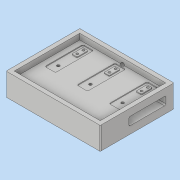
# Autodesk Inventor part: Hauptplatte
Saved by Autodesk Inventor 2018 (Build 220112000, 112)
## iProperties
Created: 2020-10-04
Part Number: Hauptplatte
Material: Generisch
Document SubType Name: Modeling
Designer: marce
Density: 1 g/cm^3
Appearance: Vorgabe
Author: marce
Autodesk Inventor part; units mm, degrees
ref_plane "YZ Plane" through (0, 0, 0) normal (1, 0, 0) x (0, 1, 0)
ref_plane "XZ Plane" through (0, 0, 0) normal (0, 1, 0) x (-1, 0, 0)
ref_plane "XY Plane" through (0, 0, 0) normal (0, 0, 1) x (1, 0, 0)
sketch "Skizze1" plane through (0, 0, 0) normal (0, 0, 1) x (1, 0, 0)
  line L0 (0, 0) -> (230, 0)
  line L1 (230, 0) -> (230, 180)
  line L2 (230, 180) -> (0, 180)
  line L3 (0, 180) -> (0, 0)
  dimension "d0" = 230
  dimension "d1" = 180
  constraints: 8 end point, 2 parallel, 1 horizontal, 1 perpendicular
  measures "d0" distance of L2.end L1.end
  measures "d1" distance of L1.end L0.end
extrude "Extrusion1" add sketch "Skizze1" along normal blind 39
sketch "Skizze2" plane through (0, 0, 39) normal (0, 0, 1) x (1, 0, 0)
  line L0 (0, 0) -> (230, 0) projected
  line L1 (230, 0) -> (230, 180) projected
  line L2 (230, 180) -> (0, 180) projected
  line L3 (0, 180) -> (0, 0) projected
  line L4 (10, 170) -> (220, 170)
  line L5 (220, 170) -> (220, 10)
  line L6 (220, 10) -> (10, 10)
  line L7 (10, 10) -> (10, 170)
  dimension "d4" = 10
  constraints: 8 end point, 3 other
  measures "d4" distance between parallel lines of L2 L4
extrude "Extrusion2" add sketch "Skizze2" along normal blind 16
sketch "Skizze3" plane through (0, 0, 39) normal (0, 0, 1) x (1, 0, 0)
  line L0 (108.5, 157.5) -> (121.5, 157.5)
  line L1 (121.5, 157.5) -> (121.5, 130.5)
  line L2 (121.5, 130.5) -> (108.5, 130.5)
  line L3 (108.5, 130.5) -> (108.5, 157.5)
  line L4 (30, 157.5) -> (43, 157.5)
  line L5 (43, 157.5) -> (43, 130.5)
  line L6 (43, 130.5) -> (30, 130.5)
  line L7 (30, 130.5) -> (30, 157.5)
  line L8 (187, 157.5) -> (200, 157.5)
  line L9 (200, 157.5) -> (200, 130.5)
  line L10 (200, 130.5) -> (187, 130.5)
  line L11 (187, 130.5) -> (187, 157.5)
  line L12 (10, 170) -> (10, 10) projected
  line L13 (220, 10) -> (220, 170) projected
  line L14 (220, 170) -> (10, 170) projected
  line L15 (23.5, 164) -> (49.5, 164)
  line L16 (49.5, 164) -> (49.5, 71)
  line L17 (49.5, 71) -> (23.5, 71)
  line L18 (23.5, 71) -> (23.5, 164)
  line L19 (102, 164) -> (128, 164)
  line L20 (128, 164) -> (128, 71)
  line L21 (128, 71) -> (102, 71)
  line L22 (102, 71) -> (102, 164)
  line L23 (180.5, 164) -> (206.5, 164)
  line L24 (206.5, 164) -> (206.5, 71)
  line L25 (206.5, 71) -> (180.5, 71)
  line L26 (180.5, 71) -> (180.5, 164)
  line L27 (220, 10) -> (220, 170) projected
  line L28 (220, 170) -> (10, 170) projected
  line L29 (10, 170) -> (10, 10) projected
  line L30 (10, 10) -> (220, 10) projected
  point P0 (0, 0)
  dimension "d7" = 27
  dimension "d8" = 13
  dimension "d9" = 27
  dimension "d10" = 13
  dimension "d11" = 27
  dimension "d12" = 13
  dimension "d13" = 20
  dimension "d14" = 20
  dimension "d15" = 65.5
  dimension "d16" = 65.5
  dimension "d17" = 12.5
  dimension "d34" = 6.5
  dimension "d35" = 6.5
  dimension "d36" = 6.5
  dimension "d37" = 6.5
  dimension "d38" = 6.5
  dimension "d39" = 6.5
  dimension "d40" = 6.5
  dimension "d42" = 93
  dimension "d43" = 93
  dimension "d44" = 93
  constraints: 48 end point, 12 parallel, 6 horizontal, 6 perpendicular, 3 collinear, 1 point on line
  measures "d7" distance of L0.end L1.end
  measures "d8" distance of L0.start L0.end
  measures "d9" distance of L4.end L5.end
  measures "d10" distance of L4.start L4.end
  measures "d11" distance of L8.end L9.end
  measures "d12" distance of L8.start L8.end
  measures "d13" distance between parallel lines of L7 L12
  measures "d14" distance between parallel lines of L13 L9
  measures "d15" distance between parallel lines of L11 L1
  measures "d16" distance between parallel lines of L5 L3
  measures "d17" distance between parallel lines of L14 L0
  measures "d34" distance between parallel lines of L18 L7
  measures "d35" distance between parallel lines of L16 L5
  measures "d36" distance between parallel lines of L3 L22
  measures "d37" distance between parallel lines of L20 L1
  measures "d38" distance between parallel lines of L26 L11
  measures "d39" distance between parallel lines of L24 L9
  measures "d40" distance between parallel lines of L23 L8
  measures "d42" distance of L21.end L19.start
  measures "d43" distance of L15.end L16.end
  measures "d44" distance of L25.end L23.start
extrude "Extrusion3" add sketch "Skizze3" along normal blind 2
sketch "Skizze4" plane through (0, 0, 41) normal (0, 0, 1) x (1, 0, 0)
  line L0 (43, 157.5) -> (30, 157.5) projected
  line L1 (30, 157.5) -> (30, 130.5) projected
  line L2 (30, 130.5) -> (43, 130.5) projected
  line L3 (43, 130.5) -> (43, 157.5) projected
  line L4 (121.5, 157.5) -> (108.5, 157.5) projected
  line L5 (108.5, 157.5) -> (108.5, 130.5) projected
  line L6 (108.5, 130.5) -> (121.5, 130.5) projected
  line L7 (121.5, 130.5) -> (121.5, 157.5) projected
  line L8 (200, 157.5) -> (187, 157.5) projected
  line L9 (187, 157.5) -> (187, 130.5) projected
  line L10 (187, 130.5) -> (200, 130.5) projected
  line L11 (200, 130.5) -> (200, 157.5) projected
  line L12 (30, 157.5) -> (36.5, 157.5)
  line L13 (36.5, 157.5) -> (36.5, 152.5)
  line L14 (36.5, 152.5) -> (30, 152.5)
  line L15 (30, 152.5) -> (30, 157.5)
  line L16 (36.5, 152.5) -> (50, 152.5)
  line L17 (50, 152.5) -> (50, 137.5)
  line L18 (50, 137.5) -> (36.5, 137.5)
  line L19 (36.5, 137.5) -> (36.5, 152.5)
  line L20 (115, 157.5) -> (120, 157.5)
  line L21 (120, 157.5) -> (120, 152.5)
  line L22 (120, 152.5) -> (115, 152.5)
  line L23 (115, 152.5) -> (115, 157.5)
  line L24 (115, 152.5) -> (121, 152.5)
  line L25 (121, 152.5) -> (121, 137.5)
  line L26 (121, 137.5) -> (115, 137.5)
  line L27 (115, 137.5) -> (115, 152.5)
  line L28 (200, 157.5) -> (187, 157.5) projected
  line L29 (193.5, 157.5) -> (198, 157.5)
  line L30 (198, 157.5) -> (198, 152.5)
  line L31 (198, 152.5) -> (193.5, 152.5)
  line L32 (193.5, 152.5) -> (193.5, 157.5)
  line L33 (193.5, 152.5) -> (200, 152.5)
  line L34 (200, 152.5) -> (200, 137.5)
  line L35 (200, 137.5) -> (193.5, 137.5)
  line L36 (193.5, 137.5) -> (193.5, 152.5)
  point P0 (0, 0)
  dimension "d20" = 15
  dimension "d21" = 5
  dimension "d29" = 5
  dimension "d30" = 15
  dimension "d31" = 5
  dimension "d32" = 15
  constraints: 48 end point, 12 parallel, 6 horizontal, 6 perpendicular, 3 midpoint, 1 point on line, 1 vertical alignment
  measures "d20" distance of L16.end L17.end
  measures "d21" distance of L12.end L13.end
  measures "d29" distance of L20.end L21.end
  measures "d30" distance of L24.end L25.end
  measures "d31" distance of L29.end L30.end
  measures "d32" distance of L33.end L34.end
hole "Bohrung1" at (36.5, 137.5, 41) at (36.5, 152.5, 41) at (115, 152.5, 41) at (115, 137.5, 41) at (193.5, 152.5, 41) at (193.5, 137.5, 41) direction (0, 0, -1) diameter 5.5 end through all
sketch "Skizze5" plane through (0, 0, 0) normal (0, 0, -1) x (-1, 0, 0)
  circle A0 centre (-193.5, 152.5) radius 2.75 projected
  circle A1 centre (-115, 152.5) radius 2.75 projected
  circle A2 centre (-36.5, 137.5) radius 2.75 projected
  circle A3 centre (-36.5, 152.5) radius 2.75 projected
  circle A4 centre (-115, 137.5) radius 2.75 projected
  circle A5 centre (-193.5, 137.5) radius 2.75 projected
  line L0 (0, 0) -> (-230, 0) projected
  line L1 (0, 180) -> (0, 0) projected
  line L2 (-230, 180) -> (0, 180) projected
  line L3 (-230, 0) -> (-230, 180) projected
  line L4 (-20, 160) -> (-20, 20)
  line L5 (-20, 20) -> (-210, 20)
  line L6 (-210, 20) -> (-210, 160)
  line L7 (-210, 160) -> (-20, 160)
  dimension "d46" = 20
  constraints: 8 end point, 3 other
  measures "d46" distance between parallel lines of L2 L7
extrude "Extrusion4" cut sketch "Skizze5" against normal blind 10 contours L4 L5 L6 L7
sketch "Skizze6" plane through (0, 0, 10) normal (0, 0, -1) x (-1, 0, 0)
  circle A0 centre (-193.5, 137.5) radius 2.75 projected
  circle A1 centre (-115, 137.5) radius 2.75 projected
  circle A2 centre (-36.5, 152.5) radius 2.75 projected
  circle A3 centre (-36.5, 137.5) radius 2.75 projected
  circle A4 centre (-115, 152.5) radius 2.75 projected
  circle A5 centre (-193.5, 152.5) radius 2.75 projected
  line L0 (-20, 160) -> (-20, 20) projected
  line L1 (-210, 160) -> (-20, 160) projected
  line L2 (-210, 20) -> (-210, 160) projected
  line L3 (-20, 20) -> (-210, 20) projected
  circle A6 centre (-193.5, 152.5) radius 2.75 projected
  circle A7 centre (-193.5, 152.5) radius 4.5
  circle A8 centre (-193.5, 137.5) radius 4.5
  circle A9 centre (-115, 152.5) radius 2.75 projected
  circle A10 centre (-115, 152.5) radius 4.5
  circle A11 centre (-115, 137.5) radius 4.5
  circle A12 centre (-36.5, 152.5) radius 2.75 projected
  circle A13 centre (-36.5, 152.5) radius 4.5
  circle A14 centre (-36.5, 137.5) radius 4.5
  point P0 (0, 0)
  dimension "d49" = 9
  dimension "d50" = 9
  dimension "d51" = 9
  dimension "d52" = 9
  dimension "d53" = 9
  dimension "d54" = 9
  constraints: 6 centre point, 6 coincident
  measures "d49" diameter of A7
  measures "d50" diameter of A8
  measures "d51" diameter of A10
  measures "d52" diameter of A11
  measures "d53" diameter of A13
  measures "d54" diameter of A14
extrude "Extrusion5" cut sketch "Skizze6" against normal blind 5.5 contours A7 | A8 | A10 | A11 | A13 | A14
sketch "Skizze7" plane through (0, 180, 0) normal (0, 1, 0) x (1, 0, 0)
  line L0 (230, 0) -> (0, 0) projected
  line L1 (0, 0) -> (0, -55) projected
  line L2 (230, -55) -> (0, -55) projected
  line L3 (230, 0) -> (230, -55) projected
  line L4 (230, -55) -> (0, -55)
  line L5 (0, -55) -> (0, -32)
  line L6 (0, -32) -> (230, -32)
  line L7 (230, -32) -> (230, -55)
  line L8 (115, -55) -> (101, -55)
  line L9 (101, -55) -> (101, -41)
  line L10 (101, -41) -> (115, -41)
  line L11 (115, -41) -> (115, -55)
  dimension "d59" = 14
  constraints: 16 end point, 4 parallel, 2 horizontal, 2 perpendicular, 1 midpoint, 1 point on line
  measures "d59" distance of L8.end L9.end
hole "Bohrung2" at (115, 180, 41) direction (0, -1, 0) diameter 10 depth 12 tip angle 118
sketch "Skizze8" plane through (0, 0, 0) normal (0, 0, -1) x (-1, 0, 0)
  line L0 (-210, 160) -> (-20, 160) projected
  line L1 (-20, 160) -> (-20, 20) projected
  line L2 (-20, 20) -> (-210, 20) projected
  line L3 (-210, 20) -> (-210, 160) projected
  line L4 (0, 0) -> (-230, 0) projected
  line L5 (0, 180) -> (0, 0) projected
  line L6 (-230, 180) -> (0, 180) projected
  line L7 (-230, 0) -> (-230, 180) projected
  line L8 (-10, 170) -> (-10, 10)
  line L9 (-10, 10) -> (-220, 10)
  line L10 (-220, 10) -> (-220, 170)
  line L11 (-220, 170) -> (-10, 170)
  dimension "d67" = 10
  dimension "d68" = 10
  constraints: 8 end point, 3 other
  measures "d67" distance between parallel lines of L6 L11
  measures "d68" distance between parallel lines of L0 L11
hole "Bohrung3" at (220, 170, 0) at (10, 170, 0) at (10, 10, 0) at (220, 10, 0) direction (0, 0, 1) diameter 6.647 depth 30 tip angle 118 thread size "M8x1.25" class "6H" standard "ISO Metric profile"
sketch "Skizze9" plane through (0, 0, 10) normal (0, 0, -1) x (-1, 0, 0)
  line L0 (-195, 121) -> (-35, 121)
  line L1 (-35, 121) -> (-35, 35)
  line L2 (-35, 35) -> (-195, 35)
  line L3 (-195, 35) -> (-195, 121)
  line L4 (-20, 160) -> (-20, 20) projected
  line L5 (-210, 20) -> (-210, 160) projected
  line L6 (-20, 20) -> (-210, 20) projected
  point P0 (0, 0)
  dimension "d76" = 15
  dimension "d77" = 15
  dimension "d78" = 15
  constraints: 8 end point, 2 parallel, 1 horizontal, 1 perpendicular
  measures "d76" distance between parallel lines of L4 L1
  measures "d77" distance between parallel lines of L5 L3
  measures "d78" distance between parallel lines of L6 L2
hole "Bohrung4" at (35, 121, 10) at (35, 35, 10) at (195, 35, 10) at (195, 121, 10) direction (0, 0, 1) diameter 6.647 depth 20 tip angle 118 thread size "M8x1.25" class "6H" standard "ISO Metric profile"
sketch "Skizze10" plane through (0, 0, 39) normal (0, 0, 1) x (1, 0, 0)
  line L0 (49.5, 71) -> (49.5, 164) projected
  line L1 (49.5, 164) -> (23.5, 164) projected
  line L2 (23.5, 164) -> (23.5, 71) projected
  line L3 (23.5, 71) -> (49.5, 71) projected
  line L4 (43, 157.5) -> (43, 130.5) projected
  line L5 (43, 130.5) -> (30, 130.5) projected
  line L6 (30, 130.5) -> (30, 157.5) projected
  line L7 (30, 157.5) -> (43, 157.5) projected
  line L8 (128, 71) -> (128, 164) projected
  line L9 (128, 164) -> (102, 164) projected
  line L10 (102, 164) -> (102, 71) projected
  line L11 (102, 71) -> (128, 71) projected
  line L12 (121.5, 157.5) -> (121.5, 130.5) projected
  line L13 (121.5, 130.5) -> (108.5, 130.5) projected
  line L14 (108.5, 130.5) -> (108.5, 157.5) projected
  line L15 (108.5, 157.5) -> (121.5, 157.5) projected
  line L16 (206.5, 71) -> (206.5, 164) projected
  line L17 (206.5, 164) -> (180.5, 164) projected
  line L18 (180.5, 164) -> (180.5, 71) projected
  line L19 (180.5, 71) -> (206.5, 71) projected
  line L20 (200, 157.5) -> (200, 130.5) projected
  line L21 (200, 130.5) -> (187, 130.5) projected
  line L22 (187, 130.5) -> (187, 157.5) projected
  line L23 (187, 157.5) -> (200, 157.5) projected
  line L24 (23.5, 71) -> (49.5, 71) projected
  line L25 (36.5, 71) -> (63, 71)
  line L26 (63, 71) -> (63, 91)
  line L27 (63, 91) -> (36.5, 91)
  line L28 (36.5, 91) -> (36.5, 71)
  line L29 (102, 71) -> (128, 71) projected
  line L30 (115, 71) -> (141, 71)
  line L31 (141, 71) -> (141, 91)
  line L32 (141, 91) -> (115, 91)
  line L33 (115, 91) -> (115, 71)
  line L34 (180.5, 71) -> (206.5, 71) projected
  line L35 (193.5, 71) -> (169, 71)
  line L36 (169, 71) -> (169, 91)
  line L37 (169, 91) -> (193.5, 91)
  line L38 (193.5, 91) -> (193.5, 71)
  point P0 (0, 0)
  dimension "d86" = 20
  constraints: 24 end point, 8 parallel, 3 horizontal, 3 midpoint, 3 perpendicular
  measures "d86" distance of L26.end L25.end
hole "Bohrung5" at (36.5, 91, 39) at (115, 91, 39) at (193.5, 91, 39) direction (0, 0, -1) diameter 6.647 end through all thread size "M8x1.25" class "6H" standard "ISO Metric profile"
sketch "Skizze11" plane through (0, 0, 10) normal (0, 0, -1) x (-1, 0, 0)
  circle A0 centre (-115, 91) radius 3.3235 projected
  circle A1 centre (-36.5, 91) radius 3.3235 projected
  circle A2 centre (-193.5, 91) radius 3.3235 projected
  circle A3 centre (-195, 35) radius 3.3235 projected
  circle A4 centre (-35, 121) radius 3.3235 projected
  circle A5 centre (-35, 35) radius 3.3235 projected
  circle A6 centre (-195, 121) radius 3.3235 projected
  circle A7 centre (-36.5, 152.5) radius 4.5 projected
  circle A8 centre (-115, 152.5) radius 4.5 projected
  circle A9 centre (-193.5, 152.5) radius 4.5 projected
  circle A10 centre (-193.5, 137.5) radius 4.5 projected
  circle A11 centre (-115, 137.5) radius 4.5 projected
  circle A12 centre (-36.5, 137.5) radius 4.5 projected
  line L0 (-20, 160) -> (-20, 20) projected
  line L1 (-210, 160) -> (-20, 160) projected
  line L2 (-210, 20) -> (-210, 160) projected
  line L3 (-20, 20) -> (-210, 20) projected
  circle A13 centre (-193.5, 91) radius 10
  circle A14 centre (-115, 91) radius 10
  circle A15 centre (-36.5, 91) radius 10
  point P0 (0, 0)
  dimension "d94" = 20
  constraints: 3 centre point, 3 coincident, 2 equal radius
  measures "d94" diameter of A13
extrude "Extrusion6" cut sketch "Skizze11" against normal blind 10 contours A13 | A14 | A15
sketch "Skizze12" plane through (230, 0, 0) normal (1, 0, 0) x (0, 0, -1)
  line L0 (-38, 70) -> (-18, 70)
  line L1 (-18, 70) -> (-18, 160)
  line L2 (-18, 160) -> (-38, 160)
  line L3 (-38, 160) -> (-38, 70)
  line L4 (0, 180) -> (-55, 180) projected
  line L5 (0, 0) -> (-55, 0) projected
  line L6 (0, 0) -> (0, 180) projected
  line L7 (-55, 0) -> (-55, 180) projected
  dimension "d99" = 90
  dimension "d100" = 20
  dimension "d101" = 20
  dimension "d102" = 70
  dimension "d103" = 18
  dimension "d104" = 17
  constraints: 8 end point, 2 parallel, 1 horizontal, 1 perpendicular
  measures "d99" distance of L2.end L0.start
  measures "d100" distance of L1.end L2.end
  measures "d101" distance between parallel lines of L4 L2
  measures "d102" distance between parallel lines of L5 L0
  measures "d103" distance between parallel lines of L6 L1
  measures "d104" distance between parallel lines of L3 L7
extrude "Extrusion7" cut sketch "Skizze12" against normal blind 25 contours L3 L2 L1 L0
fillet "Rundung3" radius 3.1 4 edges at (217.5, 70, 38) (217.5, 70, 18) (217.5, 160, 18) (217.5, 160, 38)
ref_plane "Arbeitsebene1" through (115, 0, 0) normal (1, 0, 0) x (0, 0, -1)
mirror "Spiegeln1" about plane through (115, 0, 0) normal (1, 0, 0) of "Rundung3", "Extrusion7"
fillet "Rundung2" radius 6.5 4 edges at (20, 160, 5) (210, 160, 5) (210, 20, 5) (20, 20, 5)
fillet "Rundung2" radius 2 4 edges at (230, 0, 27.5) (0, 0, 27.5) (0, 180, 27.5) (230, 180, 27.5)
fillet "Rundung1" radius 2 12 edges at (187, 130.5, 40) (200, 130.5, 40) (200, 157.5, 40) (187, 157.5, 40) (121.5, 157.5, 40) (108.5, 157.5, 40) (121.5, 130.5, 40) (108.5, 130.5, 40) (43, 130.5, 40) (30, 130.5, 40) (43, 157.5, 40) (30, 157.5, 40)
fillet "Rundung1" radius 3.5 12 edges at (23.5, 164, 40) (49.5, 164, 40) (49.5, 71, 40) (23.5, 71, 40) (102, 71, 40) (128, 71, 40) (128, 164, 40) (102, 164, 40) (180.5, 164, 40) (206.5, 164, 40) (180.5, 71, 40) (206.5, 71, 40)
equation "\"d15\" = d16"
equation "\"d42\" = d43"
equation "\"d44\" = d43"
equation "\"d67\" = d68"
equation "\"d108\" = -0.5 * d0"
